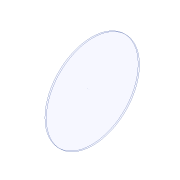
# Autodesk Inventor part: Lens
Saved by Autodesk Inventor 2020.3 (Build 243373010, 373A)
## iProperties
Created: 2020-12-03
Part Number: Lens
Material: Generic
Document SubType Name: Modeling
Designer: Yusuf
Mass: 10.107 g
Surface Area: 79.5016 cm^2
Volume: 10.107 cm^3
Density: 1 g/cm^3
Appearance: Default
Author: Yusuf
Autodesk Inventor part; units mm, degrees
ref_plane "YZ Plane" through (0, 0, 0) normal (1, 0, 0) x (0, 1, 0)
ref_plane "XZ Plane" through (0, 0, 0) normal (0, 1, 0) x (-1, 0, 0)
ref_plane "XY Plane" through (0, 0, 0) normal (0, 0, 1) x (1, 0, 0)
sketch "Sketch1" plane through (0, 0, 0) normal (0, 1, 0) x (-1, 0, 0)
  line L0 (0, 0) -> (0, 35)
  line L1 (0, 35) -> (1, 35)
  line L2 (11.6244, 0) -> (-8.6875, 0) construction
  arc A0 (1.4684, -34.9984) -> (1, 35) centre (-195.6751, -1.3169) ccw
  line L3 (0, 0) -> (4.3205, 0.0214)
  dimension "d0" = 35
  dimension "d1" = 1
  dimension "d2" = 70
  dimension "d3" = 200
  constraints: 8 end point, 3 point on circle, 1 centre point, 1 horizontal, 1 perpendicular, 1 vertical
  measures "d0" distance of L0.start L0.end
  measures "d1" distance of L0.end L1.end
  measures "d2" distance of L1.end A0.start
  measures "d3" radius of A0
revolve "Revolution1" add sketch "Sketch1" angle 360 about axis through (-11.6244, 0, 0) along (1, 0, 0)
body "Solid1"
